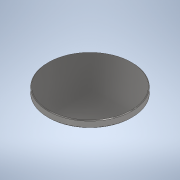
# Autodesk Inventor part: Magnet
Saved by Autodesk Inventor 2021.1 (Build 251245010, 245A)
## iProperties
Created: 2025-09-17
Material: Magnesium AZ63A
Document SubType Name: Modeling
Designer: SD
Density: 1.82745 g/cm^3
Appearance: Steel - Polished
Mass: 0.410634 g
Surface Area: 2.92655 cm^2
Volume: 0.224703 cm^3
Project: Automatic Tea Steeping mechanism
Part Number: Magnet
BOM-Mass: 0.00041
BOM-Area: 0.000
Author: SD
Title: Magnet
Autodesk Inventor part; units mm, degrees
ref_plane "YZ Plane" through (0, 0, 0) normal (1, 0, 0) x (0, 1, 0)
ref_plane "XZ Plane" through (0, 0, 0) normal (0, 1, 0) x (-1, 0, 0)
ref_plane "XY Plane" through (0, 0, 0) normal (0, 0, 1) x (1, 0, 0)
sketch "Sketch1" plane through (0, 0, 0) normal (0, 1, 0) x (-1, 0, 0)
  circle A0 centre (0, 0) radius 12.5
  dimension "d0" = 25
  constraints: 1 centre point, 1 coincident
  measures "d0" diameter of A0
extrude "Extrusion1" add sketch "Sketch1" along normal mid plane 2
chamfer "Chamfer1" distance 0.2 angle 45 2 edges at (12.5, 1, 0) (12.5, -1, 0)
body "Solid1"
